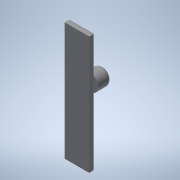
# Autodesk Inventor part: Pieza1 Pasador
Saved by Autodesk Inventor 2021.2 (Build 252289000, 289)
## iProperties
Created: 2026-08-24
Part Number: Pieza1 Pasador
Material: Generic
Document SubType Name: Modeling
Designer: nelso
Density: 1 g/cm^3
Appearance: Default
Author: nelso
Autodesk Inventor part; units mm, degrees
ref_plane "YZ Plane" through (0, 0, 0) normal (1, 0, 0) x (0, 1, 0)
ref_plane "XZ Plane" through (0, 0, 0) normal (0, 1, 0) x (-1, 0, 0)
ref_plane "XY Plane" through (0, 0, 0) normal (0, 0, 1) x (1, 0, 0)
sketch "Sketch1" plane through (0, 0, 0) normal (0, 1, 0) x (-1, 0, 0)
  line L0 (-7.5, 36) -> (7.5, 36)
  line L1 (7.5, 36) -> (7.5, -36)
  line L2 (7.5, -36) -> (-7.5, -36)
  line L3 (-7.5, -36) -> (-7.5, 36)
  line L4 (-7.5, 36) -> (7.5, -36) construction
  line L5 (7.5, 36) -> (-7.5, -36) construction
  point P0 (0, 0)
  dimension "d0" = 15
  dimension "d1" = 72
  constraints: 12 end point, 2 midpoint, 2 parallel, 1 horizontal, 1 perpendicular
  measures "d0" distance of L1.end L2.end
  measures "d1" distance of L0.end L1.end
extrude "Extrusion1" add sketch "Sketch1" along normal blind 4
fillet "Fillet1" radius 2 4 edges at (0, 4, 36) (7.5, 4, 0) (-7.5, 4, 0) (0, 4, -36)
sketch "Sketch2" plane through (0, 4, 0) normal (0, 1, 0) x (1, 0, 0)
  line L0 (7.5, 36) -> (-7.5, 36) projected
  line L1 (0, 36) -> (0, -4)
  circle A0 centre (0, -4) radius 2.5
  dimension "d7" = 40
  dimension "d8" = 5
  constraints: 2 end point, 1 centre point, 1 coincident, 1 midpoint, 1 vertical
  measures "d7" distance of L1.start L1.end
  measures "d8" diameter of A0
extrude "Extrusion2" add sketch "Sketch2" along normal blind 12
sketch "Sketch3" plane through (0, 16, 4) normal (0, 1, 0) x (1, 0, 0)
  circle A0 centre (0, 0) radius 2.5 projected
  circle A1 centre (0, 0) radius 5
  point P0 (0, 4)
  dimension "d11" = 10
  constraints: 1 centre point, 1 coincident
  measures "d11" diameter of A1
extrude "Extrusion3" add sketch "Sketch3" against normal blind 8 separate body
fillet "Fillet2" radius 2 1 edges at (-5, 16, 4)
body "Solid1"
body "Solid2"
